Autodesk Fusion 360 part; units mm, degrees
(part 2 of 2)
  spline S107 degree 3 poles (11.0485, -54.4546) (11.0559, -54.5312) (11.0709, -54.6852) (11.1724, -54.8019) (11.2235, -54.8606) knots 0 0 0 0 0.02248 0.045204 0.045204 0.045204 0.045204
  spline S108 degree 3 poles (11.2235, -54.8606) (11.2828, -54.9117) (11.4018, -55.0141) (11.5581, -55.0284) (11.6365, -55.0356) knots 0 0 0 0 0.022867 0.045862 0.045862 0.045862 0.045862
  spline S109 degree 3 poles (11.6365, -55.0356) (11.7135, -55.028) (11.8693, -55.0127) (11.989, -54.9117) (12.0495, -54.8606) knots 0 0 0 0 0.022651 0.045806 0.045806 0.045806 0.045806
  spline S110 degree 3 poles (12.0495, -54.8606) (12.0985, -54.8017) (12.1965, -54.6838) (12.2105, -54.5311) (12.2175, -54.4546) knots 0 0 0 0 0.022425 0.044871 0.044871 0.044871 0.044871
  line L520 (12.2175, -54.4546) -> (12.2175, -52.1166)
  line L521 (5.2175, -53.2856) -> (7.5485, -53.2856)
  line L522 (7.5485, -53.2856) -> (7.5485, -52.7046)
  spline S111 degree 3 poles (7.5485, -52.7046) (7.5413, -52.6278) (7.527, -52.4732) (7.4295, -52.3524) (7.3805, -52.2916) knots 0 0 0 0 0.022618 0.045479 0.045479 0.045479 0.045479
  spline S112 degree 3 poles (7.3805, -52.2916) (7.32, -52.2406) (7.2003, -52.1396) (7.0445, -52.1243) (6.9675, -52.1166) knots 0 0 0 0 0.023154 0.045806 0.045806 0.045806 0.045806
  line L523 (6.9675, -52.1166) -> (6.3795, -52.1166)
  spline S113 degree 3 poles (6.3795, -52.1166) (6.21, -52.1416) (5.8695, -52.1918) (5.8222, -52.5331) (5.7985, -52.7046) knots 0 0 0 0 0.045988 0.092418 0.092418 0.092418 0.092418
  line L524 (5.7985, -52.7046) -> (5.2175, -52.7046)
  spline S114 degree 3 poles (5.2175, -52.7046) (5.2899, -52.3639) (5.4277, -51.715) (6.073, -51.5934) (6.3795, -51.5356) knots 0 0 0 0 0.094665 0.180305 0.180305 0.180305 0.180305
  line L525 (6.3795, -51.5356) -> (7.5485, -51.5356)
  spline S115 degree 3 poles (7.5485, -51.5356) (7.7024, -51.5504) (8.0127, -51.5801) (8.2532, -51.7786) (8.3745, -51.8786) knots 0 0 0 0 0.04527 0.091283 0.091283 0.091283 0.091283
  spline S116 degree 3 poles (8.3745, -51.8786) (8.4745, -51.9987) (8.6744, -52.2386) (8.7031, -52.5494) (8.7175, -52.7046) knots 0 0 0 0 0.045723 0.091336 0.091336 0.091336 0.091336
  line L526 (8.7175, -52.7046) -> (8.7175, -54.4546)
  spline S117 degree 3 poles (8.7175, -54.4546) (8.7029, -54.6081) (8.6736, -54.9166) (8.4745, -55.1542) (8.3745, -55.2736) knots 0 0 0 0 0.045098 0.090676 0.090676 0.090676 0.090676
  spline S118 degree 3 poles (8.3745, -55.2736) (8.2532, -55.3737) (8.0127, -55.5722) (7.7024, -55.6019) (7.5485, -55.6166) knots 0 0 0 0 0.046013 0.091283 0.091283 0.091283 0.091283
  line L527 (7.5485, -55.6166) -> (6.3795, -55.6166)
  spline S119 degree 3 poles (6.3795, -55.6166) (6.2261, -55.6021) (5.9176, -55.5727) (5.6799, -55.3737) (5.5605, -55.2736) knots 0 0 0 0 0.045098 0.090677 0.090677 0.090677 0.090677
  spline S120 degree 3 poles (5.5605, -55.2736) (5.4605, -55.1542) (5.2614, -54.9166) (5.2321, -54.6081) (5.2175, -54.4546) knots 0 0 0 0 0.045579 0.090676 0.090676 0.090676 0.090676
  line L528 (5.2175, -54.4546) -> (5.2175, -53.2856)
  line L529 (7.5485, -53.8666) -> (6.3795, -53.8666)
  line L530 (6.3795, -53.8666) -> (6.3795, -54.4546)
  spline S121 degree 3 poles (6.3795, -54.4546) (6.3869, -54.5312) (6.4019, -54.6852) (6.5034, -54.8019) (6.5545, -54.8606) knots 0 0 0 0 0.02248 0.045204 0.045204 0.045204 0.045204
  spline S122 degree 3 poles (6.5545, -54.8606) (6.6138, -54.9117) (6.7328, -55.0141) (6.8891, -55.0284) (6.9675, -55.0356) knots 0 0 0 0 0.022867 0.045862 0.045862 0.045862 0.045862
  spline S123 degree 3 poles (6.9675, -55.0356) (7.0445, -55.028) (7.2003, -55.0127) (7.32, -54.9117) (7.3805, -54.8606) knots 0 0 0 0 0.022651 0.045806 0.045806 0.045806 0.045806
  spline S124 degree 3 poles (7.3805, -54.8606) (7.4295, -54.8017) (7.5275, -54.6838) (7.5415, -54.5311) (7.5485, -54.4546) knots 0 0 0 0 0.022425 0.044871 0.044871 0.044871 0.044871
  line L531 (7.5485, -54.4546) -> (7.5485, -53.8666)
  line L532 (2.2985, -55.6166) -> (1.1295, -55.6166)
  line L533 (1.1295, -55.6166) -> (1.1295, -52.1166)
  line L534 (1.1295, -52.1166) -> (0.5485, -52.1166)
  spline S125 degree 3 poles (0.5485, -52.1166) (0.4701, -52.1239) (0.3138, -52.1382) (0.1948, -52.2406) (0.1355, -52.2916) knots 0 0 0 0 0.022995 0.045862 0.045862 0.045862 0.045862
  spline S126 degree 3 poles (0.1355, -52.2916) (0.0845, -52.3522) (-0.0165, -52.4719) (-0.0319, -52.6276) (-0.0395, -52.7046) knots 0 0 0 0 0.023154 0.045806 0.045806 0.045806 0.045806
  line L535 (-0.0395, -52.7046) -> (-0.0395, -55.6166)
  line L536 (-0.0395, -55.6166) -> (-1.2015, -55.6166)
  line L537 (-1.2015, -55.6166) -> (-1.2015, -52.1166)
  line L538 (-1.2015, -52.1166) -> (-1.7895, -52.1166)
  spline S127 degree 3 poles (-1.7895, -52.1166) (-1.8661, -52.1241) (-2.02, -52.1391) (-2.1368, -52.2406) (-2.1955, -52.2916) knots 0 0 0 0 0.02248 0.045204 0.045204 0.045204 0.045204
  spline S128 degree 3 poles (-2.1955, -52.2916) (-2.2465, -52.3522) (-2.3475, -52.4719) (-2.3629, -52.6276) (-2.3705, -52.7046) knots 0 0 0 0 0.023154 0.045806 0.045806 0.045806 0.045806
  line L539 (-2.3705, -52.7046) -> (-2.3705, -55.6166)
  line L540 (-2.3705, -55.6166) -> (-3.5395, -55.6166)
  line L541 (-3.5395, -55.6166) -> (-3.5395, -53.5306)
  spline S129 degree 3 poles (-3.5395, -53.5306) (-3.5146, -53.2669) (-3.4645, -52.737) (-3.123, -52.3287) (-2.9515, -52.1236) knots 0 0 0 0 0.077531 0.155728 0.155728 0.155728 0.155728
  spline S130 degree 3 poles (-2.9515, -52.1236) (-2.7477, -51.9521) (-2.3401, -51.6092) (-1.8097, -51.5602) (-1.5445, -51.5356) knots 0 0 0 0 0.077908 0.155783 0.155783 0.155783 0.155783
  line L542 (-1.5445, -51.5356) -> (-0.0395, -51.5356)
  line L543 (-0.0395, -51.5356) -> (-0.0395, -51.7176)
  spline S131 degree 3 poles (-0.0395, -51.7176) (0.0836, -51.6646) (0.3469, -51.5512) (0.6338, -51.5411) (0.7865, -51.5356) knots 0 0 0 0 0.03986 0.085239 0.085239 0.085239 0.085239
  line L544 (0.7865, -51.5356) -> (2.2985, -51.5356)
  line L545 (2.2985, -51.5356) -> (2.2985, -55.6166)
  line L546 (-4.7015, -56.2046) -> (-4.7015, -56.7856)
  line L547 (-4.7015, -56.7856) -> (-5.8705, -56.7856)
  line L548 (-5.8705, -56.7856) -> (-5.8705, -56.2046)
  line L549 (-5.8705, -56.2046) -> (-4.7015, -56.2046)
  line L550 (-4.7015, -51.5356) -> (-4.7015, -55.6166)
  line L551 (-4.7015, -55.6166) -> (-5.8705, -55.6166)
  line L552 (-5.8705, -55.6166) -> (-5.8705, -51.5356)
  line L553 (-5.8705, -51.5356) -> (-4.7015, -51.5356)
  line L554 (-7.6205, -56.7856) -> (-8.7825, -56.7856)
  line L555 (-8.7825, -56.7856) -> (-8.7825, -55.6166)
  line L556 (-8.7825, -55.6166) -> (-9.3705, -55.6166)
  line L557 (-9.3705, -55.6166) -> (-9.3705, -55.0356)
  line L558 (-9.3705, -55.0356) -> (-8.7825, -55.0356)
  line L559 (-8.7825, -55.0356) -> (-8.7825, -52.7046)
  spline S132 degree 3 poles (-8.7825, -52.7046) (-8.7888, -52.6159) (-8.8008, -52.4463) (-8.9164, -52.3226) (-8.9715, -52.2636) knots 0 0 0 0 0.025811 0.049296 0.049296 0.049296 0.049296
  spline S133 degree 3 poles (-8.9715, -52.2636) (-9.0292, -52.221) (-9.1324, -52.1446) (-9.2588, -52.1252) (-9.3145, -52.1166) knots 0 0 0 0 0.02113 0.037814 0.037814 0.037814 0.037814
  line L560 (-9.3145, -52.1166) -> (-9.3705, -52.1166)
  line L561 (-9.3705, -52.1166) -> (-9.3705, -51.5356)
  line L562 (-9.3705, -51.5356) -> (-8.7825, -51.5356)
  spline S134 degree 3 poles (-8.7825, -51.5356) (-8.6291, -51.5502) (-8.3206, -51.5796) (-8.083, -51.7786) (-7.9635, -51.8786) knots 0 0 0 0 0.045098 0.090676 0.090676 0.090676 0.090676
  spline S135 degree 3 poles (-7.9635, -51.8786) (-7.8635, -51.9987) (-7.6636, -52.2386) (-7.6349, -52.5494) (-7.6205, -52.7046) knots 0 0 0 0 0.045723 0.091337 0.091337 0.091337 0.091337
  line L563 (-7.6205, -52.7046) -> (-7.6205, -55.0356)
  line L564 (-7.6205, -55.0356) -> (-7.0325, -55.0356)
  line L565 (-7.0325, -55.0356) -> (-7.0325, -55.6166)
  line L566 (-7.0325, -55.6166) -> (-7.6205, -55.6166)
  line L567 (-7.6205, -55.6166) -> (-7.6205, -56.7856)
  line L568 (-10.5325, -51.5356) -> (-10.5325, -56.7856)
  line L569 (-10.5325, -56.7856) -> (-11.7015, -56.7856)
  line L570 (-11.7015, -56.7856) -> (-11.7015, -55.0356)
  spline S136 degree 3 poles (-11.7015, -55.0356) (-11.7149, -55.1242) (-11.7392, -55.2849) (-11.8388, -55.4124) (-11.8835, -55.4696) knots 0 0 0 0 0.026315 0.047768 0.047768 0.047768 0.047768
  spline S137 degree 3 poles (-11.8835, -55.4696) (-11.9389, -55.5125) (-12.0561, -55.603) (-12.2044, -55.612) (-12.2825, -55.6166) knots 0 0 0 0 0.020535 0.043408 0.043408 0.043408 0.043408
  line L571 (-12.2825, -55.6166) -> (-12.8705, -55.6166)
  spline S138 degree 3 poles (-12.8705, -55.6166) (-13.0239, -55.6021) (-13.3324, -55.5727) (-13.5701, -55.3737) (-13.6895, -55.2736) knots 0 0 0 0 0.045098 0.090677 0.090677 0.090677 0.090677
  spline S139 degree 3 poles (-13.6895, -55.2736) (-13.7895, -55.1542) (-13.9886, -54.9166) (-14.0179, -54.6081) (-14.0325, -54.4546) knots 0 0 0 0 0.045578 0.090676 0.090676 0.090676 0.090676
  line L572 (-14.0325, -54.4546) -> (-14.0325, -51.5356)
  line L573 (-14.0325, -51.5356) -> (-12.8705, -51.5356)
  line L574 (-12.8705, -51.5356) -> (-12.8705, -54.4546)
  spline S140 degree 3 poles (-12.8705, -54.4546) (-12.8631, -54.5312) (-12.8481, -54.6852) (-12.7465, -54.8019) (-12.6955, -54.8606) knots 0 0 0 0 0.02248 0.045204 0.045204 0.045204 0.045204
  spline S141 degree 3 poles (-12.6955, -54.8606) (-12.6362, -54.9117) (-12.5172, -55.0141) (-12.3609, -55.0284) (-12.2825, -55.0356) knots 0 0 0 0 0.022867 0.045862 0.045862 0.045862 0.045862
  spline S142 degree 3 poles (-12.2825, -55.0356) (-12.2055, -55.028) (-12.0497, -55.0127) (-11.93, -54.9117) (-11.8695, -54.8606) knots 0 0 0 0 0.022651 0.045806 0.045806 0.045806 0.045806
  spline S143 degree 3 poles (-11.8695, -54.8606) (-11.8205, -54.8017) (-11.7225, -54.6838) (-11.7085, -54.5311) (-11.7015, -54.4546) knots 0 0 0 0 0.022425 0.044871 0.044871 0.044871 0.044871
  line L575 (-11.7015, -54.4546) -> (-11.7015, -51.5356)
  line L576 (-11.7015, -51.5356) -> (-10.5325, -51.5356)
  spline S144 degree 3 poles (-17.5395, -50.9546) (-17.571, -50.7832) (-17.6318, -50.4517) (-17.9614, -50.3943) (-18.1205, -50.3666) knots 0 0 0 0 0.047129 0.091133 0.091133 0.091133 0.091133
  line L577 (-18.1205, -50.3666) -> (-18.7015, -50.3666)
  spline S145 degree 3 poles (-18.7015, -50.3666) (-18.7799, -50.3739) (-18.9362, -50.3882) (-19.0552, -50.4906) (-19.1145, -50.5416) knots 0 0 0 0 0.022995 0.045862 0.045862 0.045862 0.045862
  spline S146 degree 3 poles (-19.1145, -50.5416) (-19.1655, -50.601) (-19.2679, -50.7199) (-19.2823, -50.8763) (-19.2895, -50.9546) knots 0 0 0 0 0.022866 0.045862 0.045862 0.045862 0.045862
  line L578 (-19.2895, -50.9546) -> (-19.2895, -52.1166)
  spline S147 degree 3 poles (-19.2895, -52.1166) (-19.2517, -51.9473) (-19.1794, -51.6233) (-18.8559, -51.564) (-18.7015, -51.5356) knots 0 0 0 0 0.047223 0.090343 0.090343 0.090343 0.090343
  line L579 (-18.7015, -51.5356) -> (-18.1205, -51.5356)
  spline S148 degree 3 poles (-18.1205, -51.5356) (-17.9666, -51.5504) (-17.6563, -51.5801) (-17.4158, -51.7786) (-17.2945, -51.8786) knots 0 0 0 0 0.045269 0.091282 0.091282 0.091282 0.091282
  spline S149 degree 3 poles (-17.2945, -51.8786) (-17.1945, -51.9987) (-16.9946, -52.2386) (-16.9659, -52.5494) (-16.9515, -52.7046) knots 0 0 0 0 0.045723 0.091337 0.091337 0.091337 0.091337
  line L580 (-16.9515, -52.7046) -> (-16.9515, -55.6166)
  line L581 (-16.9515, -55.6166) -> (-18.1205, -55.6166)
  line L582 (-18.1205, -55.6166) -> (-18.1205, -52.7046)
  spline S150 degree 3 poles (-18.1205, -52.7046) (-18.1277, -52.6278) (-18.142, -52.4732) (-18.2395, -52.3524) (-18.2885, -52.2916) knots 0 0 0 0 0.022618 0.045479 0.045479 0.045479 0.045479
  spline S151 degree 3 poles (-18.2885, -52.2916) (-18.349, -52.2406) (-18.4687, -52.1396) (-18.6245, -52.1243) (-18.7015, -52.1166) knots 0 0 0 0 0.023155 0.045806 0.045806 0.045806 0.045806
  spline S152 degree 3 poles (-18.7015, -52.1166) (-18.7799, -52.1239) (-18.9362, -52.1382) (-19.0552, -52.2406) (-19.1145, -52.2916) knots 0 0 0 0 0.022995 0.045862 0.045862 0.045862 0.045862
  spline S153 degree 3 poles (-19.1145, -52.2916) (-19.1655, -52.3522) (-19.2665, -52.4719) (-19.2819, -52.6276) (-19.2895, -52.7046) knots 0 0 0 0 0.023154 0.045806 0.045806 0.045806 0.045806
  line L583 (-19.2895, -52.7046) -> (-19.2895, -55.6166)
  line L584 (-19.2895, -55.6166) -> (-20.4515, -55.6166)
  line L585 (-20.4515, -55.6166) -> (-20.4515, -50.9546)
  spline S154 degree 3 poles (-20.4515, -50.9546) (-20.4369, -50.8012) (-20.4076, -50.4927) (-20.2085, -50.2551) (-20.1085, -50.1356) knots 0 0 0 0 0.045098 0.090676 0.090676 0.090676 0.090676
  spline S155 degree 3 poles (-20.1085, -50.1356) (-19.9893, -50.0336) (-19.7528, -49.8311) (-19.4431, -49.8007) (-19.2895, -49.7856) knots 0 0 0 0 0.045877 0.091009 0.091009 0.091009 0.091009
  line L586 (-19.2895, -49.7856) -> (-18.1205, -49.7856)
  spline S156 degree 3 poles (-18.1205, -49.7856) (-17.8137, -49.8434) (-17.1676, -49.9651) (-17.0259, -50.6139) (-16.9515, -50.9546) knots 0 0 0 0 0.085805 0.180669 0.180669 0.180669 0.180669
  line L587 (-16.9515, -50.9546) -> (-17.5395, -50.9546)
  line L588 (-22.7895, -55.6166) -> (-23.9585, -55.6166)
  spline S157 degree 3 poles (-23.9585, -55.6166) (-24.1119, -55.6021) (-24.4204, -55.5727) (-24.6581, -55.3737) (-24.7775, -55.2736) knots 0 0 0 0 0.045098 0.090677 0.090677 0.090677 0.090677
  spline S158 degree 3 poles (-24.7775, -55.2736) (-24.8775, -55.1542) (-25.0766, -54.9166) (-25.1059, -54.6081) (-25.1205, -54.4546) knots 0 0 0 0 0.045579 0.090677 0.090677 0.090677 0.090677
  line L589 (-25.1205, -54.4546) -> (-25.1205, -52.7046)
  spline S159 degree 3 poles (-25.1205, -52.7046) (-25.1058, -52.5508) (-25.076, -52.2405) (-24.8775, -51.9999) (-24.7775, -51.8786) knots 0 0 0 0 0.04527 0.091282 0.091282 0.091282 0.091282
  spline S160 degree 3 poles (-24.7775, -51.8786) (-24.6581, -51.7786) (-24.4204, -51.5796) (-24.1119, -51.5502) (-23.9585, -51.5356) knots 0 0 0 0 0.045579 0.090677 0.090677 0.090677 0.090677
  line L590 (-23.9585, -51.5356) -> (-22.7895, -51.5356)
  spline S161 degree 3 poles (-22.7895, -51.5356) (-22.6356, -51.5504) (-22.3253, -51.5801) (-22.0848, -51.7786) (-21.9635, -51.8786) knots 0 0 0 0 0.045269 0.091282 0.091282 0.091282 0.091282
  spline S162 degree 3 poles (-21.9635, -51.8786) (-21.8635, -51.9987) (-21.6636, -52.2386) (-21.6349, -52.5494) (-21.6205, -52.7046) knots 0 0 0 0 0.045723 0.091337 0.091337 0.091337 0.091337
  line L591 (-21.6205, -52.7046) -> (-21.6205, -54.4546)
  spline S163 degree 3 poles (-21.6205, -54.4546) (-21.6351, -54.6081) (-21.6644, -54.9166) (-21.8635, -55.1542) (-21.9635, -55.2736) knots 0 0 0 0 0.045098 0.090677 0.090677 0.090677 0.090677
  spline S164 degree 3 poles (-21.9635, -55.2736) (-22.0848, -55.3737) (-22.3253, -55.5722) (-22.6356, -55.6019) (-22.7895, -55.6166) knots 0 0 0 0 0.046013 0.091282 0.091282 0.091282 0.091282
  line L592 (-22.7895, -54.4546) -> (-22.7895, -52.7046)
  spline S165 degree 3 poles (-22.7895, -52.7046) (-22.7967, -52.6278) (-22.811, -52.4732) (-22.9085, -52.3524) (-22.9575, -52.2916) knots 0 0 0 0 0.022618 0.045479 0.045479 0.045479 0.045479
  spline S166 degree 3 poles (-22.9575, -52.2916) (-23.018, -52.2406) (-23.1377, -52.1396) (-23.2935, -52.1243) (-23.3705, -52.1166) knots 0 0 0 0 0.023155 0.045806 0.045806 0.045806 0.045806
  spline S167 degree 3 poles (-23.3705, -52.1166) (-23.4489, -52.1239) (-23.6052, -52.1382) (-23.7242, -52.2406) (-23.7835, -52.2916) knots 0 0 0 0 0.022995 0.045862 0.045862 0.045862 0.045862
  spline S168 degree 3 poles (-23.7835, -52.2916) (-23.8345, -52.3522) (-23.9355, -52.4719) (-23.9509, -52.6276) (-23.9585, -52.7046) knots 0 0 0 0 0.023154 0.045806 0.045806 0.045806 0.045806
  line L593 (-23.9585, -52.7046) -> (-23.9585, -54.4546)
  spline S169 degree 3 poles (-23.9585, -54.4546) (-23.951, -54.5312) (-23.9361, -54.6852) (-23.8345, -54.8019) (-23.7835, -54.8606) knots 0 0 0 0 0.02248 0.045203 0.045203 0.045203 0.045203
  spline S170 degree 3 poles (-23.7835, -54.8606) (-23.7242, -54.9117) (-23.6052, -55.0141) (-23.4489, -55.0284) (-23.3705, -55.0356) knots 0 0 0 0 0.022866 0.045862 0.045862 0.045862 0.045862
  spline S171 degree 3 poles (-23.3705, -55.0356) (-23.2935, -55.028) (-23.1377, -55.0127) (-23.018, -54.9117) (-22.9575, -54.8606) knots 0 0 0 0 0.022651 0.045806 0.045806 0.045806 0.045806
  spline S172 degree 3 poles (-22.9575, -54.8606) (-22.9085, -54.8017) (-22.8105, -54.6838) (-22.7965, -54.5311) (-22.7895, -54.4546) knots 0 0 0 0 0.022425 0.044871 0.044871 0.044871 0.044871
  line L594 (-29.7895, -55.6166) -> (-29.7895, -51.5356)
  line L595 (-29.7895, -51.5356) -> (-28.6275, -51.5356)
  line L596 (-28.6275, -51.5356) -> (-28.6275, -52.1166)
  spline S173 degree 3 poles (-28.6275, -52.1166) (-28.5897, -51.9473) (-28.5174, -51.6233) (-28.1939, -51.564) (-28.0395, -51.5356) knots 0 0 0 0 0.047223 0.090343 0.090343 0.090343 0.090343
  line L597 (-28.0395, -51.5356) -> (-27.4585, -51.5356)
  spline S174 degree 3 poles (-27.4585, -51.5356) (-27.3046, -51.5504) (-26.9943, -51.5801) (-26.7538, -51.7786) (-26.6325, -51.8786) knots 0 0 0 0 0.045269 0.091282 0.091282 0.091282 0.091282
  spline S175 degree 3 poles (-26.6325, -51.8786) (-26.5325, -51.9987) (-26.3326, -52.2386) (-26.3039, -52.5494) (-26.2895, -52.7046) knots 0 0 0 0 0.045723 0.091337 0.091337 0.091337 0.091337
  line L598 (-26.2895, -52.7046) -> (-26.2895, -55.6166)
  line L599 (-26.2895, -55.6166) -> (-27.4585, -55.6166)
  line L600 (-27.4585, -55.6166) -> (-27.4585, -52.7046)
  spline S176 degree 3 poles (-27.4585, -52.7046) (-27.4657, -52.6278) (-27.48, -52.4732) (-27.5775, -52.3524) (-27.6265, -52.2916) knots 0 0 0 0 0.022618 0.045479 0.045479 0.045479 0.045479
  spline S177 degree 3 poles (-27.6265, -52.2916) (-27.687, -52.2406) (-27.8067, -52.1396) (-27.9625, -52.1243) (-28.0395, -52.1166) knots 0 0 0 0 0.023155 0.045806 0.045806 0.045806 0.045806
  spline S178 degree 3 poles (-28.0395, -52.1166) (-28.1179, -52.1239) (-28.2742, -52.1382) (-28.3932, -52.2406) (-28.4525, -52.2916) knots 0 0 0 0 0.022995 0.045862 0.045862 0.045862 0.045862
  spline S179 degree 3 poles (-28.4525, -52.2916) (-28.5035, -52.3522) (-28.6045, -52.4719) (-28.6199, -52.6276) (-28.6275, -52.7046) knots 0 0 0 0 0.023154 0.045806 0.045806 0.045806 0.045806
  line L601 (-28.6275, -52.7046) -> (-28.6275, -55.6166)
  line L602 (-28.6275, -55.6166) -> (-29.7895, -55.6166)
  line L603 (-31.5465, -55.0356) -> (-31.5465, -56.7856)
  line L604 (-31.5465, -56.7856) -> (-32.1275, -56.7856)
  line L605 (-32.1275, -56.7856) -> (-32.1275, -55.0356)
  line L606 (-32.1275, -55.0356) -> (-31.5465, -55.0356)
  line L607 (-32.7085, -55.0356) -> (-32.7085, -56.7856)
  line L608 (-32.7085, -56.7856) -> (-33.2965, -56.7856)
  line L609 (-33.2965, -56.7856) -> (-33.2965, -55.0356)
  line L610 (-33.2965, -55.0356) -> (-32.7085, -55.0356)
extrude "Extrude5" cut sketch "Sketch4" against normal blind 20 contours L4 L5 L6 L7 L8 L9 L10 L11 L12 L13 L14 L15 L16 L17 L18 L19 L20 L21 L22 L23 L24 L25 L26 L27 L28 L29 L30 L31 L32 L33 L34 L35 L36 L37 L38 L39 L40 L41 L42 L43 L44 L45 L46 L47 L48 L49 L50 L51 L52 L53 L54 L55 L56 L57 L58 L59 L60 L61 L62 L63 L64 L65 L66 L67 L68 L69 L70 L71 L72 L73 L74 L75 L76 L77 L78 L79 L80 L81 L82 L83 L84 L85 L86 L87 L88 L89 L90 L91 L92 L93 L94 L95 L96 L97 L98 L99 L100 L101 L102 L103 L104 L105 L106 L107 L108 L109 L110 L111 L112 L113 L114 L115 L116 L117 L118 L119 L120 L121 L122 L123 L124 L125 | L126 L127 L128 L129 L130 L131 L132 L133 L134 L135 L136 L137 L138 L139 L140 L141 L142 L143 L144 L145 L146 L147 L148 L149 L150 L151 L152 L153 L154 L155 L156 L157 L158 L159 L160 L161 L162 L163 L164 L165 L166 L167 L168 L169 L170 L171 L172 L173 L174 L175 L176 L177 L178 L179 L180 L181 L182 L183 L184 L185 L186 L187 L188 L189 L190 L191 L192 L193 L194 L195 L196 L197 L198 L199 L200 L201 L202 L203 L204 L205 L206 L207 L208 L209 L210 L211 L212 L213 L214 L215 L216 L217 L218 L219 L220 L221 L222 L223 L224 L225 L226 L227 L228 L229 L230 L231 L232 L233 L234 L235 L236 L237 L238 L239 L240 L241 L242 L243 L244 L245 L246 L247 L248 L249 L250 L251 L252 L253 L254 L255 L256 | L257 L258 L259 L260 L261 L262 L263 L264 L265 L266 L267 L268 L269 L270 L271 L272 L273 L274 L275 L276 L277 L278 L279 L280 L281 L282 L283 L284 L285 L286 L287 L288 L289 L290 L291 L292 L293 L294 L295 L296 L297 L298 L299 L300 L301 L302 L303 L304 L305 L306 L307 L308 L309 L310 L311 L312 L313 L314 L315 L316 L317 L318 L319 L320 L321 L322 L323 L324 L325 L326 L327 L328 L329 L330 L331 L332 L333 L334 L335 L336 L337 L338 L339 L340 L341 L342 L343 L344 L345 L346 L347 L348 L349 L350 L351 L352 L353 L354 L355 L356 L357 L358 L359 L360 L361 L362 L363 L364 L365 L366 L367 L368 L369 L370 L371 L372 L373 L374 L375 L376 L377 L378 L379 L380 L381 L382 L383 L384 L385 L386 L387 L388 L389 L390
extrude "Extrude6" cut sketch "Sketch4" against normal blind 1 contours L391 L392 L393 L394 | L395 L396 L397 L398 | L399 L400 L401 L402 L403 L404 L405 L406 L407 L408 L409 L410 | L411 S0 S1 L412 S2 L413 S3 L414 S4 S5 L415 L416 L417 S6 L418 S7 S8 S9 S10 L419 | S17 L422 S18 S19 L423 S20 L424 S21 S22 L425 L426 L427 S23 S24 S25 S26 L428 L429 L430 S27 S28 L431 S29 L432 | L433 L434 L435 L436 L437 L438 S30 S31 L439 L440 L441 S32 S33 L442 L443 L444 L445 L446 | L447 L448 L449 S34 S35 L450 S36 S37 L451 L452 L453 S38 S39 S40 S41 L454 L455 | L456 L457 S42 S43 L458 S44 L459 S45 L460 S46 S47 L461 S48 S49 L462 S50 S51 L463 | L467 L468 L469 S56 S57 L470 S58 S59 L471 L472 L473 S60 S61 S62 S63 L474 L475 | L476 L477 S64 S65 L478 S66 L479 S67 L480 S68 S69 L481 S70 S71 L482 S72 S73 L483 | L487 S78 S79 L488 S80 L489 S81 L490 S82 S83 L491 L492 L493 S84 L494 S85 S86 S87 S88 L495 | L498 L499 L500 L501 L502 L503 S95 S96 L504 L505 L506 S97 S98 L507 L508 L509 L510 L511 | L512 L513 L514 S99 S100 L515 S101 S102 L516 S103 S104 L517 | L521 L522 S111 S112 L523 S113 L524 S114 L525 S115 S116 L526 S117 S118 L527 S119 S120 L528 | L532 L533 L534 S125 S126 L535 L536 L537 L538 S127 S128 L539 L540 L541 S129 S130 L542 L543 S131 L544 L545 | L546 L547 L548 L549 | L550 L551 L552 L553 | L554 L555 L556 L557 L558 L559 S132 S133 L560 L561 L562 S134 S135 L563 L564 L565 L566 L567 | L568 L569 L570 S136 S137 L571 S138 S139 L572 L573 L574 S140 S141 S142 S143 L575 L576 | S144 L577 S145 S146 L578 S147 L579 S148 S149 L580 L581 L582 S150 S151 S152 S153 L583 L584 L585 S154 S155 L586 S156 L587 | L588 S157 S158 L589 S159 S160 L590 S161 S162 L591 S163 S164 | L594 L595 L596 S173 L597 S174 S175 L598 L599 L600 S176 S177 S178 S179 L601 L602 | L603 L604 L605 L606 | L607 L608 L609 L610
extrude "Extrude3" [suppressed]
extrude "Extrude4" [suppressed]
fillet "Fillet1" [suppressed]
extrude "Extrude2" [suppressed]
combine "Combine1" [suppressed]
combine "Combine1'" [suppressed] in component "Component"
sketch "Sketch3" plane through (0, 0, 5) normal (0, 0, 1) x (-1, 0, 0)
  arc A0 (75, -65) -> (77, -63) centre (75, -63) ccw
  line L0 (77, -63) -> (77, -5)
  arc A1 (77, -5) -> (75, -3) centre (75, -5) ccw
  line L1 (75, -3) -> (-39, -3)
  arc A2 (-39, -3) -> (-41, -5) centre (-39, -5) ccw
  line L2 (-41, -5) -> (-41, -63)
  arc A3 (-41, -63) -> (-39, -65) centre (-39, -63) ccw
  line L3 (-39, -65) -> (75, -65)
  line L4 (23.3704, -16.139) -> (-35.8533, -16.139) construction
  line L5 (-35.8533, -16.139) -> (-35.8533, -26.139) construction
  line L6 (-35.8533, -26.139) -> (23.3704, -26.139) construction
  line L7 (23.3704, -26.139) -> (23.3704, -16.139) construction
  line L8 (37.3383, -30.107) -> (-25.152, -30.107) construction
  line L9 (-25.152, -30.107) -> (-25.152, -40.107) construction
  line L10 (-25.152, -40.107) -> (37.3383, -40.107) construction
  line L11 (37.3383, -40.107) -> (37.3383, -30.107) construction
  constraint perpendicular L4 L5
  constraint parallel L4 L6
  constraint parallel L5 L7
  constraint perpendicular L8 L9
  constraint parallel L8 L10
  constraint parallel L9 L11
